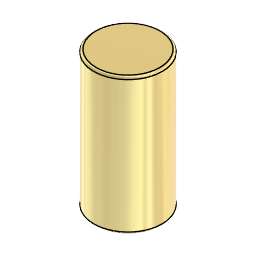
CYLINDER (Autodesk Fusion 360 design; units mm, degrees)
part number: 2025-09-14-11-53-35-571
Autodesk Fusion 360 part; units mm, degrees
sketch "草图1" plane through (0, 0, 0) normal (0, 0, 1) x (1, 0, 0)
  circle A0 centre (0, 0) radius 15
  dimension "d1" = 30
  constraint coincident A0.centre origin
  measures "d1" diameter of A0
extrude "拉伸1" add sketch "草图1" along normal blind 60
fillet "圆角1" radius 1 1 faces at (3.8315, 5.6199, 60)
fillet "圆角2" radius 1 4 faces at (-2.3333, 2.3068, 60) (-11.9131, 9.0239, 59.3271) (14.9814, -0.7477, 39.3333) (3.8315, 5.6199, 0)
equation "d1 = dia"
equation "dia = 30 mm"
equation "h = 60 mm"
equation "d4 = h"
named bodies: "Cylinder"
